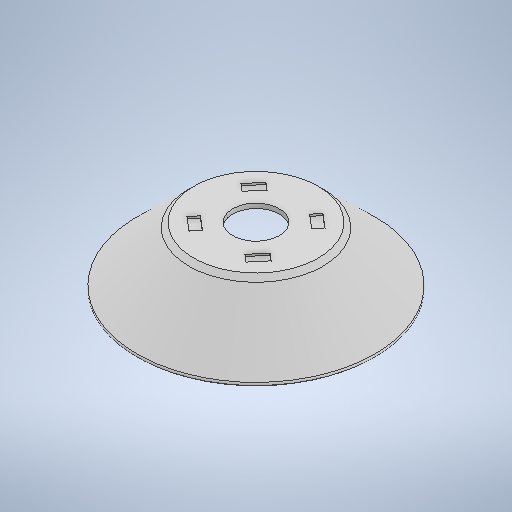
# Autodesk Inventor part: Back Cover
Saved by Autodesk Inventor 2026.2 (Build 302298000, 298)
## iProperties
Created: 2026-01-18
Part Number: Back Cover
Material: Generic
Document SubType Name: Modeling
Designer: daryu
Density: 1 g/cm^3
Appearance: Default
Author: daryu
Autodesk Inventor part; units mm, degrees
ref_plane "YZ Plane" through (0, 0, 0) normal (1, 0, 0) x (0, 1, 0)
ref_plane "XZ Plane" through (0, 0, 0) normal (0, 1, 0) x (-1, 0, 0)
ref_plane "XY Plane" through (0, 0, 0) normal (0, 0, 1) x (1, 0, 0)
sketch "Sketch1" plane through (0, 0, 0) normal (1, 0, 0) x (0, 1, 0)
  line L0 (8.865, -31.4879) -> (23.3, -16.54)
  line L1 (23.3, -16.54) -> (23.2885, -19.3531)
  line L2 (10.1754, -32.9308) -> (23.2885, -19.3531)
  arc A0 (8.865, -31.4879) -> (10.1754, -32.9308) centre (54.9627, 9.0608) ccw
  line L3 (9.5145, -32.2145) -> (23.2942, -17.9465)
  line L4 (0, 0) -> (23.3, 0)
  line L5 (0, 0) -> (26.462, 0)
  line L6 (23.3, 0) -> (23.3, -16.54)
  line L7 (23.3, -16.54) -> (15.7759, -24.3314)
  line L8 (23.2885, -19.3531) -> (27.5047, -14.9875)
  line L9 (23.3, 0) -> (24.534, 0)
  line L10 (24.534, 0) -> (24.534, -16.6628)
  line L11 (23.2942, -17.9465) -> (24.534, -16.6628)
  dimension "d0" = 23.3
  dimension "d1" = 16.54
  dimension "d2" = 18.8761
  dimension "d3" = 20.78
  dimension "d4" = 61.3938
  dimension "d5" = 2.8131
  dimension "d6" = 136
  dimension "d17" = 1.9491
  dimension "d18" = 16.6628
  dimension "d19" = 1.928
  dimension "d20" = 4.3656
  dimension "d21" = 7.1565
  constraints: 24 end point, 3 point on circle, 2 collinear, 2 horizontal, 2 parallel, 2 vertical, 1 centre point, 1 midpoint, 1 point on line
  measures "d0" distance of L4.start L4.end
  measures "d1" distance of L4.end L0.end
  measures "d2" distance of L2.start L1.end
  measures "d3" distance of L0.end L0.start
  measures "d4" radius of A0
  measures "d5" distance of L0.end L1.end
  measures "d6" angle of L7 L6
  measures "d17" distance of L2.start L0.start
  measures "d18" distance of L9.end L10.end
  measures "d19" distance of L9.end L5.end
  measures "d20" vertical distance of L1.end L8.end
  measures "d21" vertical distance of L0.start L7.end
revolve "Revolution1" add sketch "Sketch1" angle 360 about axis through (0, 0, 0) along (0, 1, 0) contours L0 L1 L3 A0 | L6 L5 L10 L11 L1
sketch "Sketch2" plane through (0, 24.534, 0) normal (0, 1, 0) x (1, 0, 0)
  circle A0 centre (0, 0) radius 6.25
  dimension "d8" = 12.5
  constraints: 1 centre point, 1 coincident
  measures "d8" diameter of A0
hole "Hole1" at (0, 24.534, 0) direction (0, -1, 0) diameter 12.5 depth 2
fillet "Fillet1" radius 0.5 1 edges at (0, 9.5145, 32.2145)
sketch "Sketch5" plane through (0, 24.534, 0) normal (0, 1, 0) x (1, 0, 0)
  line L0 (-5.9666, 8.9326) -> (-7.9148, 10.5784)
  line L1 (-7.9148, 10.5784) -> (-10.9871, 6.9417)
  line L2 (-10.9871, 6.9417) -> (-9.0388, 5.2958)
  line L3 (-9.0388, 5.2958) -> (-5.9666, 8.9326)
  line L4 (-6.9417, -10.9871) -> (-5.2958, -9.0388)
  line L5 (-8.9326, -5.9666) -> (-10.5784, -7.9148)
  line L6 (-10.5784, -7.9148) -> (-6.9417, -10.9871)
  line L7 (-5.2958, -9.0388) -> (-8.9326, -5.9666)
  line L8 (10.9871, -6.9417) -> (9.0388, -5.2958)
  line L9 (5.9666, -8.9326) -> (7.9148, -10.5784)
  line L10 (7.9148, -10.5784) -> (10.9871, -6.9417)
  line L11 (9.0388, -5.2958) -> (5.9666, -8.9326)
  line L12 (6.9417, 10.9871) -> (5.2958, 9.0388)
  line L13 (8.9326, 5.9666) -> (10.5784, 7.9148)
  line L14 (10.5784, 7.9148) -> (6.9417, 10.9871)
  line L15 (5.2958, 9.0388) -> (8.9326, 5.9666)
  point P0 (0, 0)
  point P1 (0, 0)
  point P2 (-10.0129, 6.1188)
  point P3 (-6.1188, -10.0129)
  point P4 (10.0129, -6.1188)
  point P5 (6.1188, 10.0129)
  dimension "d28" = 4.7607
  dimension "d29" = 2.5504
  dimension "d30" = 5.2958
  dimension "d31" = 9.0388
  dimension "d32" = 6.1188
  dimension "d33" = 360
  constraints: 32 end point, 2 parallel, 1 coincident, 1 midpoint, 1 perpendicular, 37 other
  measures "d28" distance of L3.start L0.start
  measures "d29" distance of L0.start L0.end
  measures "d30" vertical distance of point (0, 0) L3.start
  measures "d31" horizontal distance of point (0, 0) L3.start
  measures "d32" vertical distance of point (0, 0) point (-10.013, 6.119)
extrude "Extrusion1" cut sketch "Sketch5" against normal blind 0.5
body "Solid1"
